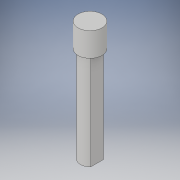
# Autodesk Inventor part: Gear_Leverage
Saved by Autodesk Inventor 2019 (Build 230136000, 136)
## iProperties
Created: 2019-05-21
Part Number: Gear_Leverage
Material: Generic
Document SubType Name: Modeling
Designer: Jorian Brusind
Density: 1 g/cm^3
Appearance: Default
Author: Jorian Brusind
Autodesk Inventor part; units mm, degrees
ref_plane "YZ Plane" through (0, 0, 0) normal (1, 0, 0) x (0, 1, 0)
ref_plane "XZ Plane" through (0, 0, 0) normal (0, 1, 0) x (-1, 0, 0)
ref_plane "XY Plane" through (0, 0, 0) normal (0, 0, 1) x (1, 0, 0)
sketch "Sketch1" plane through (0, 0, 0) normal (0, 1, 0) x (-1, 0, 0)
  circle A0 centre (0, 0) radius 5
  line L0 (0, 0) -> (3.5355, -3.5355)
  line L1 (0, 0) -> (5, 0) construction
  dimension "d0" = 10
  dimension "d1" = 5
  dimension "d2" = 45
  constraints: 4 end point, 1 centre point, 1 coincident, 1 equal length, 1 horizontal
  measures "d0" diameter of A0
  measures "d1" distance of L0.start L0.end
  measures "d2" angle of L0 L1
extrude "Extrusion1" add sketch "Sketch1" along normal blind 5
sketch "Sketch3" plane through (0, 5, 0) normal (0, 1, 0) x (1, 0, 0)
  circle A0 centre (0, 0) radius 5
  dimension "d47" = 10
  constraints: 1 centre point, 1 coincident
  measures "d47" diameter of A0
sketch "Sketch4" plane through (0, 0, 0) normal (0, -1, 0) x (1, 0, 0)
  circle A0 centre (0, 0) radius 4
  line L0 (0, 0) -> (3, 0)
  line L1 (3, 0) -> (3, -2.6458)
  line L2 (3, 0) -> (3, 2.6458)
  line L3 (0, 0) -> (-3, 0)
  line L4 (-3, 0) -> (-3, -2.6458)
  line L5 (-3, 0) -> (-3, 2.6458)
  dimension "d33" = 8
  dimension "d34" = 3
  dimension "d35" = 3
  constraints: 12 end point, 4 point on circle, 3 point on line, 2 perpendicular, 1 centre point, 1 coincident, 1 horizontal
  measures "d33" diameter of A0
  measures "d34" distance of L0.start L0.end
  measures "d35" distance of L0.start L3.end
extrude "Extrusion4" add sketch "Sketch4" along normal blind 40 contours L2 L0 L3 L5 A0 | A0 L4 L3 L0 L1
extrude "Extrusion6" add sketch "Sketch3" along normal blind 5
body "Solid1"
